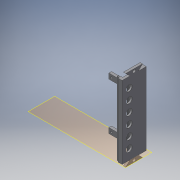
# Autodesk Inventor part: TopFrame
Saved by Autodesk Inventor 2016 SP2 (Build 200236200, 236)
## iProperties
Created: 2018-06-21
Part Number: TopFrame
Material: Generisch
Document SubType Name: Modeling
Designer: Nils
Density: 1 g/cm^3
Appearance: Vorgabe
Author: Nils
Autodesk Inventor part; units mm, degrees
ref_plane "YZ Plane" through (0, 0, 0) normal (1, 0, 0) x (0, 1, 0)
ref_plane "XZ Plane" through (0, 0, 0) normal (0, 1, 0) x (-1, 0, 0)
ref_plane "XY Plane" through (0, 0, 0) normal (0, 0, 1) x (1, 0, 0)
ref_plane "Arbeitsebene1" through (0, 0, 0) normal (0, 0, 1) x (1, 0, 0)
sketch "Skizze1" plane through (0, 0, 0) normal (0, 0, 1) x (1, 0, 0)
  line L0 (159.5, 1) -> (168.5, 1) projected
  line L1 (159.5, 0) -> (159.5, 1) projected
  line L2 (161, 0) -> (161, -17) projected
  line L3 (159.5, 0) -> (161, 0) projected
  line L4 (168.5, -14) -> (168.5, 1) projected
  line L5 (159.5, -17) -> (161, -17) projected
  line L6 (159.5, -17) -> (159.5, -17.5) projected
  line L7 (161, -19) -> (159.5, -17.5) projected
  line L8 (168.5, -6) -> (168.5, -38) projected
  line L9 (168.5, -45) -> (168.5, -30) projected
  line L10 (168.5, -45) -> (161, -45) projected
  line L11 (159.5, -22.5) -> (157.9, -22.5) construction
  line L12 (157.9, -22.5) -> (157.9, -40.5) construction
  line L13 (157.9, -40.5) -> (159.5, -40.5) construction
  line L14 (159.5, -40.5) -> (159.5, -22.5) construction
  line L15 (167.9, -24) -> (164, -24) construction
  line L16 (164, -24) -> (164, -39) construction
  line L17 (164, -39) -> (167.9, -39) construction
  line L18 (167.9, -39) -> (167.9, -24) construction
  line L19 (167.9, -25.5) -> (168.5, -25.5) construction
  line L20 (168.5, -25.5) -> (168.5, -37.5) construction
  line L21 (168.5, -37.5) -> (167.9, -37.5) construction
  line L22 (167.9, -37.5) -> (167.9, -25.5) construction
  line L23 (164, -31.5) -> (167.9, -31.5) construction
  line L24 (168.5, -31.5) -> (167.9, -31.5) construction
  line L25 (164, -31.5) -> (159.5, -31.5) construction
  line L26 (159.5, -22.5) -> (160.5261, -23.5261) construction
  line L27 (159.5, -22.5) -> (160.9511, -22.5) construction
  line L28 (164, -31.5) -> (167.9, -31.5) construction
  line L29 (159.5, -22.5) -> (158.7, -21.7) construction
  line L30 (158.7, -21.7) -> (156.9, -23.5) construction
  line L31 (156.9, -23.5) -> (156.9, -19) construction
  line L32 (156.9, -19) -> (161, -19) construction
  line L33 (157.9, -40.5) -> (156.9, -39.5) construction
  line L34 (158.7, -41.3) -> (160.5, -39.5) construction
  line L35 (160.5, -39.5) -> (164, -39.5) construction
  line L36 (164, -39.5) -> (164, -39) construction
  line L37 (160.5261, -23.5261) -> (164, -23.5261) construction
  line L38 (164, -23.5261) -> (164, -24) construction
  line L39 (157.9, -40.5) -> (158.7, -41.3) construction
  line L40 (156.9, -39.5) -> (156.9, -43) construction
  line L41 (161, -45) -> (161, -43)
  line L42 (161, -43) -> (156.9, -43)
  line L43 (161, -19) -> (156.9, -19)
  line L44 (156.9, -19) -> (156.9, -23.5)
  line L45 (156.9, -23.5) -> (158.7, -21.7)
  line L46 (158.7, -21.7) -> (160.5261, -23.5261)
  line L47 (160.5261, -23.5261) -> (164, -23.5261)
  line L48 (164, -23.5261) -> (164, -24)
  line L49 (164, -24) -> (164, -39.5)
  line L50 (164, -39.5) -> (160.5, -39.5)
  line L51 (160.5, -39.5) -> (158.7, -41.3)
  line L52 (158.7, -41.3) -> (156.9, -39.5)
  line L53 (156.9, -39.5) -> (156.9, -43)
  point P0 (0, 0)
  dimension "d0" = 0.6
  dimension "d2" = 6.1
  dimension "d4" = 12
  dimension "d5" = 15
  dimension "d6" = 1.6
  dimension "d7" = 4.5
  dimension "d8" = 18
  dimension "d9" = 45
  dimension "d10" = 1.0261
  dimension "d11" = 6
  dimension "d12" = 1
  dimension "d13" = 0.8
  dimension "d14" = 0.8
  dimension "d15" = 1
  dimension "d16" = 1
  dimension "d17" = 0.8
  dimension "d18" = 1
  dimension "d19" = 2
  dimension "d69" = 3.9
  constraints: 87 end point, 13 perpendicular, 7 parallel, 6 horizontal, 6 midpoint, 5 collinear, 5 point on line, 3 vertical, 1 equal length
  measures "d0" distance between parallel lines of L18 L8
  measures "d2" distance between parallel lines of L16 L12
  measures "d4" distance between parallel lines of L21 L19
  measures "d5" distance of L15.end L16.end
  measures "d6" distance between parallel lines of L12 L14
  measures "d7" distance between parallel lines of L8 L16
  measures "d8" distance of L11.end L12.end
  measures "d9" angle of L26 L27
  measures "d10" horizontal distance of L26.end L11.start
  measures "d11" distance between parallel lines of L10 L17
  measures "d12" horizontal distance of L13.end L34.end
  measures "d13" distance from line of L12 L29.end
  measures "d14" horizontal distance of L11.end L29.end
  measures "d15" horizontal distance of L11.end L30.end
  measures "d16" horizontal distance of L33.end L12.end
  measures "d17" horizontal distance of L34.start L13.end
  measures "d18" horizontal distance of L34.end L13.end
  measures "d19" distance of L10.end L41.end
  measures "d69" distance between parallel lines of L16 L22
extrude "Extrusion1" add sketch "Skizze1" along normal blind 138.8
sketch "Skizze2" plane through (168.5, -45, 0) normal (1, 0, 0) x (0, 0, -1)
  line L0 (0, 46) -> (-138.8, 46) construction
  line L1 (-69.4, 46) -> (-69.4, 0) construction
  circle A0 centre (4, 23) radius 1.75 projected
  line L2 (0, 15) -> (0, 31) projected
  line L3 (8, 7) -> (0, 15) projected
  line L4 (8, 39) -> (8, 7) projected
  line L5 (0, 31) -> (8, 39) projected
  circle A1 centre (-142.8, 23) radius 1.75
  line L6 (-138.8, 15) -> (-138.8, 31)
  line L7 (-146.8, 7) -> (-138.8, 15)
  line L8 (-146.8, 39) -> (-146.8, 7)
  line L9 (-138.8, 31) -> (-146.8, 39)
  point P0 (0, 45)
  constraints: 5 symmetric about line, 2 end point, 1 midpoint, 1 vertical, 1 other
extrude "Extrusion2" add sketch "Skizze2" against normal blind 4.4
sketch "Skizze3" plane through (168.5, 1, 138.8) normal (1, 0, 0) x (0, 0, -1)
  circle A0 centre (142.8, -23) radius 1.75 projected
  circle A1 centre (-4, -23) radius 1.75 projected
  circle A2 centre (142.8, -23) radius 3
  circle A3 centre (-4, -23) radius 3
  point P0 (138.8, -1)
  dimension "d24" = 6
  dimension "d25" = 6
  constraints: 2 centre point, 2 coincident
  measures "d24" diameter of A2
  measures "d25" diameter of A3
extrude "Extrusion3" cut sketch "Skizze3" against normal blind 3.5
sketch "Skizze4" plane through (156.9, -23.5, 0) normal (-1, 0, 0) x (0, 0, 1)
  line L0 (109.4004, 2.5) -> (119.4004, 2.5) projected
  line L1 (119.4004, 2.5) -> (119.4004, -2.5) projected
  line L2 (119.4004, -2.5) -> (109.4004, -2.5) projected
  line L3 (109.4004, -2.5) -> (109.4004, 2.5) projected
  line L4 (19.4004, 2.5) -> (29.4004, 2.5) projected
  line L5 (29.4004, 2.5) -> (29.4004, -2.5) projected
  line L6 (29.4004, -2.5) -> (19.4004, -2.5) projected
  line L7 (19.4004, -2.5) -> (19.4004, 2.5) projected
  point P0 (0, 23.5)
extrude "Extrusion4" add sketch "Skizze4" along normal blind 32.65
chamfer "Fase1" distance 2.5 angle 45 2 edges at (156.9, -26, 114.4004) (156.9, -26, 24.4004)
sketch "Skizze5" plane through (124.25, -26, 29.4004) normal (0, -1, 0) x (1, 0, 0)
  circle A0 centre (5, -5) radius 1.75
  circle A1 centre (5, 85) radius 1.75
  line L0 (32.65, 0) -> (0, 0) projected
  line L1 (0, -10) -> (0, 0) projected
  line L2 (0, 80) -> (0, 90) projected
  line L3 (32.65, 90) -> (0, 90) projected
  point P0 (-124.25, -29.4004)
  dimension "d33" = 3.5
  dimension "d34" = 3.5
  dimension "d35" = 5
  dimension "d36" = 5
  dimension "d37" = 5
  dimension "d38" = 5
  constraints: 2 centre point
  measures "d33" diameter of A0
  measures "d34" diameter of A1
  measures "d35" distance from line of L0 A0.centre
  measures "d36" distance from line of L1 A0.centre
  measures "d37" distance from line of L2 A1.centre
  measures "d38" distance from line of L3 A1.centre
extrude "Extrusion5" cut sketch "Skizze5" against normal blind 36.75
sketch "Skizze7" plane through (156.9, -21, 119.4004) normal (0, 1, 0) x (1, 0, 0)
  circle A0 centre (-27.65, 5) radius 1.75 construction
  circle A1 centre (-27.65, 95) radius 1.75 construction
  line L0 (-29.3243, 7.9) -> (-25.9757, 7.9)
  line L1 (-25.9757, 7.9) -> (-24.3014, 5)
  line L2 (-24.3014, 5) -> (-25.9757, 2.1)
  line L3 (-25.9757, 2.1) -> (-29.3243, 2.1)
  line L4 (-29.3243, 2.1) -> (-30.9986, 5)
  line L5 (-30.9986, 5) -> (-29.3243, 7.9)
  line L6 (-29.3243, 97.9) -> (-25.9757, 97.9)
  line L7 (-25.9757, 97.9) -> (-24.3014, 95)
  line L8 (-24.3014, 95) -> (-25.9757, 92.1)
  line L9 (-25.9757, 92.1) -> (-29.3243, 92.1)
  line L10 (-29.3243, 92.1) -> (-30.9986, 95)
  line L11 (-30.9986, 95) -> (-29.3243, 97.9)
  point P0 (-156.9, 119.4004)
  dimension "d41" = 5.8
  dimension "d43" = 5.8
  constraints: 24 end point, 2 coincident, 2 horizontal, 26 other
  measures "d41" distance between parallel lines of L6 L9
  measures "d43" distance between parallel lines of L0 L3
extrude "Extrusion6" cut sketch "Skizze7" against normal blind 2.5
chamfer "Fase2" distance 2 angle 45 2 edges at (156.9, -21, 114.4004) (156.9, -21, 24.4004)
sketch "Skizze8" plane through (164, -39.5, 0) normal (-1, 0, 0) x (0, 0, 1)
  line L0 (0, 9.5) -> (0, -5.5) construction
  line L1 (0, 0) -> (0, 15.9739) construction
  line L2 (0, 7.987) -> (138.8, 7.987) construction
  line L3 (138.8, -5.5) -> (138.8, 9.5) construction
  circle A0 centre (19.4, 7.987) radius 7.5
  circle A1 centre (39.4, 7.987) radius 7.5
  circle A2 centre (59.4, 7.987) radius 7.5
  circle A3 centre (79.4, 7.987) radius 7.5
  circle A4 centre (99.4, 7.987) radius 7.5
  circle A5 centre (119.4, 7.987) radius 7.5
  point P0 (0, 39.5)
  dimension "d49" = 15
  dimension "d50" = 19.4
  dimension "d53" = 20
  dimension "d58" = 19.4
  constraints: 6 centre point, 3 point on line, 2 end point, 2 horizontal, 1 midpoint, 10 other
  measures "d49" diameter of A0
  measures "d50" distance of A0.centre L2.start
  measures "d53" distance of A0.centre A1.centre
  measures "d58" distance from line of L3 A5.centre
extrude "Extrusion7" cut sketch "Skizze8" against normal blind 3.9
sketch "Skizze9" plane through (167.9, -31.513, 19.4) normal (-1, 0, 0) x (0, 0, 1)
  circle A0 centre (0, 0) radius 7.5 projected
  circle A1 centre (20, 0) radius 7.5 projected
  circle A2 centre (40, 0) radius 7.5 projected
  circle A3 centre (60, 0) radius 7.5 projected
  circle A4 centre (80, 0) radius 7.5 projected
  circle A5 centre (100, 0) radius 7.5 projected
  circle A6 centre (0, 0) radius 6
  circle A7 centre (20, 0) radius 6
  circle A8 centre (40, 0) radius 6
  circle A9 centre (60, 0) radius 6
  circle A10 centre (80, 0) radius 6
  circle A11 centre (100, 0) radius 6
  point P0 (-19.4, 31.513)
  dimension "d61" = 12
  dimension "d62" = 12
  dimension "d63" = 12
  dimension "d64" = 12
  dimension "d65" = 12
  dimension "d66" = 12
  constraints: 6 centre point, 6 coincident
  measures "d61" diameter of A6
  measures "d62" diameter of A7
  measures "d63" diameter of A8
  measures "d64" diameter of A9
  measures "d65" diameter of A10
  measures "d66" diameter of A11
extrude "Extrusion8" cut sketch "Skizze9" against normal blind 3.9 contours A6 | A7 | A8 | A9 | A10 | A11
equation "\"d25\" = d24"
